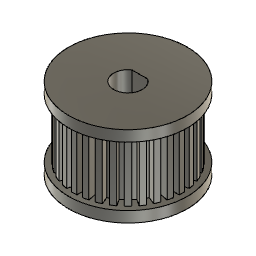
pulley2032 (Autodesk Fusion 360 design; units mm, degrees)
Autodesk Fusion 360 part; units mm, degrees
note: some values were not read from the file. Set by a fixed rule: which sketch regions a step uses.
sketch "Sketch1" plane through (0, 0, 0) normal (0, 0, 1) x (1, 0, 0)
  line L0 (0, 0) -> (0, 8.5) construction
  line L1 (0.5, 8.5) -> (-0.5, 8.5)
  line L2 (-0.5, 8.5) -> (-0.5, 10)
  line L3 (-0.5, 10) -> (0.5, 10)
  line L4 (0.5, 10) -> (0.5, 8.5)
  line L5 (-1.4605, 9.9054) -> (-1.1679, 8.4342)
  line L6 (-2.4413, 9.7103) -> (-1.4605, 9.9054)
  line L7 (-2.1487, 8.2391) -> (-2.4413, 9.7103)
  line L8 (-3.3649, 9.4301) -> (-2.7909, 8.0443)
  line L9 (-4.2888, 9.0475) -> (-3.3649, 9.4301)
  line L10 (-3.7147, 7.6616) -> (-4.2888, 9.0475)
  line L11 (-5.14, 8.5925) -> (-4.3066, 7.3453)
  line L12 (-5.9714, 8.0369) -> (-5.14, 8.5925)
  line L13 (-5.1381, 6.7897) -> (-5.9714, 8.0369)
  line L14 (-6.7175, 7.4246) -> (-5.6569, 6.364)
  line L15 (-7.4246, 6.7175) -> (-6.7175, 7.4246)
  line L16 (-6.364, 5.6569) -> (-7.4246, 6.7175)
  line L17 (-8.0369, 5.9714) -> (-6.7897, 5.1381)
  line L18 (-8.5925, 5.14) -> (-8.0369, 5.9714)
  line L19 (-7.3453, 4.3066) -> (-8.5925, 5.14)
  line L20 (-9.0475, 4.2888) -> (-7.6616, 3.7147)
  line L21 (-9.4301, 3.3649) -> (-9.0475, 4.2888)
  line L22 (-8.0443, 2.7909) -> (-9.4301, 3.3649)
  line L23 (-9.7103, 2.4413) -> (-8.2391, 2.1487)
  line L24 (-9.9054, 1.4605) -> (-9.7103, 2.4413)
  line L25 (-8.4342, 1.1679) -> (-9.9054, 1.4605)
  line L26 (-10, 0.5) -> (-8.5, 0.5)
  line L27 (-10, -0.5) -> (-10, 0.5)
  line L28 (-8.5, -0.5) -> (-10, -0.5)
  line L29 (-9.9054, -1.4605) -> (-8.4342, -1.1679)
  line L30 (-9.7103, -2.4413) -> (-9.9054, -1.4605)
  line L31 (-8.2391, -2.1487) -> (-9.7103, -2.4413)
  line L32 (-9.4301, -3.3649) -> (-8.0443, -2.7909)
  line L33 (-9.0475, -4.2888) -> (-9.4301, -3.3649)
  line L34 (-7.6616, -3.7147) -> (-9.0475, -4.2888)
  line L35 (-8.5925, -5.14) -> (-7.3453, -4.3066)
  line L36 (-8.0369, -5.9714) -> (-8.5925, -5.14)
  line L37 (-6.7897, -5.1381) -> (-8.0369, -5.9714)
  line L38 (-7.4246, -6.7175) -> (-6.364, -5.6569)
  line L39 (-6.7175, -7.4246) -> (-7.4246, -6.7175)
  line L40 (-5.6569, -6.364) -> (-6.7175, -7.4246)
  line L41 (-5.9714, -8.0369) -> (-5.1381, -6.7897)
  line L42 (-5.14, -8.5925) -> (-5.9714, -8.0369)
  line L43 (-4.3066, -7.3453) -> (-5.14, -8.5925)
  line L44 (-4.2888, -9.0475) -> (-3.7147, -7.6616)
  line L45 (-3.3649, -9.4301) -> (-4.2888, -9.0475)
  line L46 (-2.7909, -8.0443) -> (-3.3649, -9.4301)
  line L47 (-2.4413, -9.7103) -> (-2.1487, -8.2391)
  line L48 (-1.4605, -9.9054) -> (-2.4413, -9.7103)
  line L49 (-1.1679, -8.4342) -> (-1.4605, -9.9054)
  line L50 (-0.5, -10) -> (-0.5, -8.5)
  line L51 (0.5, -10) -> (-0.5, -10)
  line L52 (0.5, -8.5) -> (0.5, -10)
  line L53 (1.4605, -9.9054) -> (1.1679, -8.4342)
  line L54 (2.4413, -9.7103) -> (1.4605, -9.9054)
  line L55 (2.1487, -8.2391) -> (2.4413, -9.7103)
  line L56 (3.3649, -9.4301) -> (2.7909, -8.0443)
  line L57 (4.2888, -9.0475) -> (3.3649, -9.4301)
  line L58 (3.7147, -7.6616) -> (4.2888, -9.0475)
  line L59 (5.14, -8.5925) -> (4.3066, -7.3453)
  line L60 (5.9714, -8.0369) -> (5.14, -8.5925)
  line L61 (5.1381, -6.7897) -> (5.9714, -8.0369)
  line L62 (6.7175, -7.4246) -> (5.6569, -6.364)
  line L63 (7.4246, -6.7175) -> (6.7175, -7.4246)
  line L64 (6.364, -5.6569) -> (7.4246, -6.7175)
  line L65 (8.0369, -5.9714) -> (6.7897, -5.1381)
  line L66 (8.5925, -5.14) -> (8.0369, -5.9714)
  line L67 (7.3453, -4.3066) -> (8.5925, -5.14)
  line L68 (9.0475, -4.2888) -> (7.6616, -3.7147)
  line L69 (9.4301, -3.3649) -> (9.0475, -4.2888)
  line L70 (8.0443, -2.7909) -> (9.4301, -3.3649)
  line L71 (9.7103, -2.4413) -> (8.2391, -2.1487)
  line L72 (9.9054, -1.4605) -> (9.7103, -2.4413)
  line L73 (8.4342, -1.1679) -> (9.9054, -1.4605)
  line L74 (10, -0.5) -> (8.5, -0.5)
  line L75 (10, 0.5) -> (10, -0.5)
  line L76 (8.5, 0.5) -> (10, 0.5)
  line L77 (9.9054, 1.4605) -> (8.4342, 1.1679)
  line L78 (9.7103, 2.4413) -> (9.9054, 1.4605)
  line L79 (8.2391, 2.1487) -> (9.7103, 2.4413)
  line L80 (9.4301, 3.3649) -> (8.0443, 2.7909)
  line L81 (9.0475, 4.2888) -> (9.4301, 3.3649)
  line L82 (7.6616, 3.7147) -> (9.0475, 4.2888)
  line L83 (8.5925, 5.14) -> (7.3453, 4.3066)
  line L84 (8.0369, 5.9714) -> (8.5925, 5.14)
  line L85 (6.7897, 5.1381) -> (8.0369, 5.9714)
  line L86 (7.4246, 6.7175) -> (6.364, 5.6569)
  line L87 (6.7175, 7.4246) -> (7.4246, 6.7175)
  line L88 (5.6569, 6.364) -> (6.7175, 7.4246)
  line L89 (5.9714, 8.0369) -> (5.1381, 6.7897)
  line L90 (5.14, 8.5925) -> (5.9714, 8.0369)
  line L91 (4.3066, 7.3453) -> (5.14, 8.5925)
  line L92 (4.2888, 9.0475) -> (3.7147, 7.6616)
  line L93 (3.3649, 9.4301) -> (4.2888, 9.0475)
  line L94 (2.7909, 8.0443) -> (3.3649, 9.4301)
  line L95 (2.4413, 9.7103) -> (2.1487, 8.2391)
  line L96 (1.4605, 9.9054) -> (2.4413, 9.7103)
  line L97 (1.1679, 8.4342) -> (1.4605, 9.9054)
  circle A0 centre (0, 0) radius 8.5147
  circle A1 centre (0, 0) radius 11
  dimension "d2" = 1
  dimension "d3" = 1.5
  dimension "d5" = 360
  dimension "d11" = 10
  dimension "d13" = 22
  constraint coincident L0.start A0.centre
  constraint vertical L0
  constraint horizontal L1
  constraint vertical L2
  constraint horizontal L3
  constraint vertical L4
  constraint collinear L0.end L1.start L1.end
  constraint midpoint L0.end L1
  constraint coincident L1.start A0
  measures "d2" distance of L2.end L3.end
  measures "d3" distance of L1.start L3.end
  measures "d11" distance of L0.start L3
  measures "d13" diameter of A1
extrude "Extrude1" add sketch "Sketch1" along normal blind 15 contours L1 A0 | L2 L3 L4 A0 | L1 A0 | L95 L96 L97 A0 | L5 L6 L7 A0 | L92 L93 L94 A0 | L8 L9 L10 A0 | L89 L90 L91 A0 | L11 L12 L13 A0 | L86 L87 L88 A0 | L14 L15 L16 A0 | L83 L84 L85 A0 | L17 L18 L19 A0 | L80 L81 L82 A0 | L20 L21 L22 A0 | L77 L78 L79 A0 | L23 L24 L25 A0 | L74 L75 L76 A0 | L26 L27 L28 A0 | L29 L30 L31 A0 | L71 L72 L73 A0 | L32 L33 L34 A0 | L68 L69 L70 A0 | L35 L36 L37 A0 | L65 L66 L67 A0 | L38 L39 L40 A0 | L62 L63 L64 A0 | L41 L42 L43 A0 | L59 L60 L61 A0 | L44 L45 L46 A0 | L56 L57 L58 A0 | L47 L48 L49 A0 | L53 L54 L55 A0 | L50 L51 L52 A0
sketch "Sketch2" plane through (0, 0, 15) normal (0, 0, 1) x (-1, 0, 0)
  arc A0 (-8.2391, -2.1487) -> (-8.0443, -2.7909) centre (0, 0) ccw
  line L0 (-8.0443, -2.7909) -> (-9.4301, -3.3649)
  line L1 (-9.4301, -3.3649) -> (-9.0475, -4.2888)
  line L2 (-9.0475, -4.2888) -> (-7.6616, -3.7147)
  arc A1 (-7.6616, -3.7147) -> (-7.3453, -4.3066) centre (0, 0) ccw
  line L3 (-7.3453, -4.3066) -> (-8.5925, -5.14)
  line L4 (-8.5925, -5.14) -> (-8.0369, -5.9714)
  line L5 (-8.0369, -5.9714) -> (-6.7897, -5.1381)
  arc A2 (-6.7897, -5.1381) -> (-6.364, -5.6569) centre (0, 0) ccw
  line L6 (-6.364, -5.6569) -> (-7.4246, -6.7175)
  line L7 (-7.4246, -6.7175) -> (-6.7175, -7.4246)
  line L8 (-6.7175, -7.4246) -> (-5.6569, -6.364)
  arc A3 (-5.6569, -6.364) -> (-5.1381, -6.7897) centre (0, 0) ccw
  line L9 (-5.1381, -6.7897) -> (-5.9714, -8.0369)
  line L10 (-5.9714, -8.0369) -> (-5.14, -8.5925)
  line L11 (-5.14, -8.5925) -> (-4.3066, -7.3453)
  arc A4 (-4.3066, -7.3453) -> (-3.7147, -7.6616) centre (0, 0) ccw
  line L12 (-3.7147, -7.6616) -> (-4.2888, -9.0475)
  line L13 (-4.2888, -9.0475) -> (-3.3649, -9.4301)
  line L14 (-3.3649, -9.4301) -> (-2.7909, -8.0443)
  arc A5 (-2.7909, -8.0443) -> (-2.1487, -8.2391) centre (0, 0) ccw
  line L15 (-2.1487, -8.2391) -> (-2.4413, -9.7103)
  line L16 (-2.4413, -9.7103) -> (-1.4605, -9.9054)
  line L17 (-1.4605, -9.9054) -> (-1.1679, -8.4342)
  arc A6 (-1.1679, -8.4342) -> (-0.5, -8.5) centre (0, 0) ccw
  line L18 (-0.5, -8.5) -> (-0.5, -10)
  line L19 (-0.5, -10) -> (0.5, -10)
  line L20 (0.5, -10) -> (0.5, -8.5)
  arc A7 (0.5, -8.5) -> (1.1679, -8.4342) centre (0, 0) ccw
  line L21 (1.1679, -8.4342) -> (1.4605, -9.9054)
  line L22 (1.4605, -9.9054) -> (2.4413, -9.7103)
  line L23 (2.4413, -9.7103) -> (2.1487, -8.2391)
  arc A8 (2.1487, -8.2391) -> (2.7909, -8.0443) centre (0, 0) ccw
  line L24 (2.7909, -8.0443) -> (3.3649, -9.4301)
  line L25 (3.3649, -9.4301) -> (4.2888, -9.0475)
  line L26 (4.2888, -9.0475) -> (3.7147, -7.6616)
  arc A9 (3.7147, -7.6616) -> (4.3066, -7.3453) centre (0, 0) ccw
  line L27 (4.3066, -7.3453) -> (5.14, -8.5925)
  line L28 (5.14, -8.5925) -> (5.9714, -8.0369)
  line L29 (5.9714, -8.0369) -> (5.1381, -6.7897)
  arc A10 (5.1381, -6.7897) -> (5.6569, -6.364) centre (0, 0) ccw
  line L30 (5.6569, -6.364) -> (6.7175, -7.4246)
  line L31 (6.7175, -7.4246) -> (7.4246, -6.7175)
  line L32 (7.4246, -6.7175) -> (6.364, -5.6569)
  arc A11 (6.364, -5.6569) -> (6.7897, -5.1381) centre (0, 0) ccw
  line L33 (6.7897, -5.1381) -> (8.0369, -5.9714)
  line L34 (8.0369, -5.9714) -> (8.5925, -5.14)
  line L35 (8.5925, -5.14) -> (7.3453, -4.3066)
  arc A12 (7.3453, -4.3066) -> (7.6616, -3.7147) centre (0, 0) ccw
  line L36 (7.6616, -3.7147) -> (9.0475, -4.2888)
  line L37 (9.0475, -4.2888) -> (9.4301, -3.3649)
  line L38 (9.4301, -3.3649) -> (8.0443, -2.7909)
  arc A13 (8.0443, -2.7909) -> (8.2391, -2.1487) centre (0, 0) ccw
  line L39 (8.2391, -2.1487) -> (9.7103, -2.4413)
  line L40 (9.7103, -2.4413) -> (9.9054, -1.4605)
  line L41 (9.9054, -1.4605) -> (8.4342, -1.1679)
  arc A14 (8.4342, -1.1679) -> (8.5, -0.5) centre (0, 0) ccw
  line L42 (8.5, -0.5) -> (10, -0.5)
  line L43 (10, -0.5) -> (10, 0.5)
  line L44 (10, 0.5) -> (8.5, 0.5)
  arc A15 (8.5, 0.5) -> (8.4342, 1.1679) centre (0, 0) ccw
  line L45 (8.4342, 1.1679) -> (9.9054, 1.4605)
  line L46 (9.9054, 1.4605) -> (9.7103, 2.4413)
  line L47 (9.7103, 2.4413) -> (8.2391, 2.1487)
  arc A16 (8.2391, 2.1487) -> (8.0443, 2.7909) centre (0, 0) ccw
  line L48 (8.0443, 2.7909) -> (9.4301, 3.3649)
  line L49 (9.4301, 3.3649) -> (9.0475, 4.2888)
  line L50 (9.0475, 4.2888) -> (7.6616, 3.7147)
  arc A17 (7.6616, 3.7147) -> (7.3453, 4.3066) centre (0, 0) ccw
  line L51 (7.3453, 4.3066) -> (8.5925, 5.14)
  line L52 (8.5925, 5.14) -> (8.0369, 5.9714)
  line L53 (8.0369, 5.9714) -> (6.7897, 5.1381)
  arc A18 (6.7897, 5.1381) -> (6.364, 5.6569) centre (0, 0) ccw
  line L54 (6.364, 5.6569) -> (7.4246, 6.7175)
  line L55 (7.4246, 6.7175) -> (6.7175, 7.4246)
  line L56 (6.7175, 7.4246) -> (5.6569, 6.364)
  arc A19 (5.6569, 6.364) -> (5.1381, 6.7897) centre (0, 0) ccw
  line L57 (5.1381, 6.7897) -> (5.9714, 8.0369)
  line L58 (5.9714, 8.0369) -> (5.14, 8.5925)
  line L59 (5.14, 8.5925) -> (4.3066, 7.3453)
  arc A20 (4.3066, 7.3453) -> (3.7147, 7.6616) centre (0, 0) ccw
  line L60 (3.7147, 7.6616) -> (4.2888, 9.0475)
  line L61 (4.2888, 9.0475) -> (3.3649, 9.4301)
  line L62 (3.3649, 9.4301) -> (2.7909, 8.0443)
  arc A21 (2.7909, 8.0443) -> (2.1487, 8.2391) centre (0, 0) ccw
  line L63 (2.1487, 8.2391) -> (2.4413, 9.7103)
  line L64 (2.4413, 9.7103) -> (1.4605, 9.9054)
  line L65 (1.4605, 9.9054) -> (1.1679, 8.4342)
  arc A22 (1.1679, 8.4342) -> (0.5, 8.5) centre (0, 0) ccw
  line L66 (0.5, 8.5) -> (0.5, 10)
  line L67 (0.5, 10) -> (-0.5, 10)
  line L68 (-0.5, 10) -> (-0.5, 8.5)
  arc A23 (-0.5, 8.5) -> (-1.1679, 8.4342) centre (0, 0) ccw
  line L69 (-1.1679, 8.4342) -> (-1.4605, 9.9054)
  line L70 (-1.4605, 9.9054) -> (-2.4413, 9.7103)
  line L71 (-2.4413, 9.7103) -> (-2.1487, 8.2391)
  arc A24 (-2.1487, 8.2391) -> (-2.7909, 8.0443) centre (0, 0) ccw
  line L72 (-2.7909, 8.0443) -> (-3.3649, 9.4301)
  line L73 (-3.3649, 9.4301) -> (-4.2888, 9.0475)
  line L74 (-4.2888, 9.0475) -> (-3.7147, 7.6616)
  arc A25 (-3.7147, 7.6616) -> (-4.3066, 7.3453) centre (0, 0) ccw
  line L75 (-4.3066, 7.3453) -> (-5.14, 8.5925)
  line L76 (-5.14, 8.5925) -> (-5.9714, 8.0369)
  line L77 (-5.9714, 8.0369) -> (-5.1381, 6.7897)
  arc A26 (-5.1381, 6.7897) -> (-5.6569, 6.364) centre (0, 0) ccw
  line L78 (-5.6569, 6.364) -> (-6.7175, 7.4246)
  line L79 (-6.7175, 7.4246) -> (-7.4246, 6.7175)
  line L80 (-7.4246, 6.7175) -> (-6.364, 5.6569)
  arc A27 (-6.364, 5.6569) -> (-6.7897, 5.1381) centre (0, 0) ccw
  line L81 (-6.7897, 5.1381) -> (-8.0369, 5.9714)
  line L82 (-8.0369, 5.9714) -> (-8.5925, 5.14)
  line L83 (-8.5925, 5.14) -> (-7.3453, 4.3066)
  arc A28 (-7.3453, 4.3066) -> (-7.6616, 3.7147) centre (0, 0) ccw
  line L84 (-7.6616, 3.7147) -> (-9.0475, 4.2888)
  line L85 (-9.0475, 4.2888) -> (-9.4301, 3.3649)
  line L86 (-9.4301, 3.3649) -> (-8.0443, 2.7909)
  arc A29 (-8.0443, 2.7909) -> (-8.2391, 2.1487) centre (0, 0) ccw
  line L87 (-8.2391, 2.1487) -> (-9.7103, 2.4413)
  line L88 (-9.7103, 2.4413) -> (-9.9054, 1.4605)
  line L89 (-9.9054, 1.4605) -> (-8.4342, 1.1679)
  arc A30 (-8.4342, 1.1679) -> (-8.5, 0.5) centre (0, 0) ccw
  line L90 (-8.5, 0.5) -> (-10, 0.5)
  line L91 (-10, 0.5) -> (-10, -0.5)
  line L92 (-10, -0.5) -> (-8.5, -0.5)
  arc A31 (-8.5, -0.5) -> (-8.4342, -1.1679) centre (0, 0) ccw
  line L93 (-8.4342, -1.1679) -> (-9.9054, -1.4605)
  line L94 (-9.9054, -1.4605) -> (-9.7103, -2.4413)
  line L95 (-9.7103, -2.4413) -> (-8.2391, -2.1487)
  line L96 (1.4773, -2.2) -> (-1.4773, -2.2)
  arc A32 (1.4773, -2.2) -> (-1.4773, -2.2) centre (0, 0) ccw
  dimension "d8" = 5.3
  dimension "d12" = 2.2
  constraint concentric A0 A32
  constraint horizontal L96
  measures "d8" diameter of A32
  measures "d12" distance of A0.centre L96
extrude "Extrude2" cut sketch "Sketch2" against normal through all contours L96 A32
extrude "Extrude3" add sketch "Sketch1" along normal blind 2
extrude "Extrude4" add sketch "Sketch1" against normal blind 2 from surface at 15
